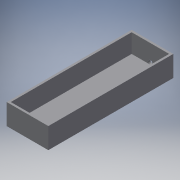
# Autodesk Inventor part: Trough
Saved by Autodesk Inventor 2019 (Build 230136000, 136)
## iProperties
Created: 2019-11-13
Part Number: Trough
Material: Generic
Document SubType Name: Modeling
Designer: Administrator
Density: 1 g/cm^3
Appearance: Default
Author: Administrator
Autodesk Inventor part; units mm, degrees
ref_plane "YZ Plane" through (0, 0, 0) normal (1, 0, 0) x (0, 1, 0)
ref_plane "XZ Plane" through (0, 0, 0) normal (0, 1, 0) x (-1, 0, 0)
ref_plane "XY Plane" through (0, 0, 0) normal (0, 0, 1) x (1, 0, 0)
sketch "Sketch1" plane through (0, 0, 0) normal (0, 1, 0) x (-1, 0, 0)
  line L0 (254, 762) -> (-254, 762)
  line L1 (-254, 762) -> (-254, -762)
  line L2 (-254, -762) -> (254, -762)
  line L3 (254, -762) -> (254, 762)
  line L4 (254, 762) -> (-254, -762) construction
  line L5 (-254, 762) -> (254, -762) construction
  point P0 (0, 0)
  dimension "d0" = 508
  dimension "d1" = 1524
  constraints: 12 end point, 2 midpoint, 2 parallel, 1 horizontal, 1 perpendicular
  measures "d0" distance of L2.end L1.end
  measures "d1" distance of L1.end L0.end
extrude "Extrusion1" add sketch "Sketch1" along normal blind 254
sketch "Sketch2" plane through (0, 254, 0) normal (0, 1, 0) x (1, 0, 0)
  line L0 (-254, -762) -> (254, -762) projected
  line L1 (254, 762) -> (-254, 762)
  line L2 (-254, 762) -> (-254, -762)
  line L3 (-254, -762) -> (254, -762)
  line L4 (254, -762) -> (254, 762)
  line L5 (254, 762) -> (-254, -762) construction
  line L6 (-254, 762) -> (254, -762) construction
  line L7 (0, -762) -> (0, -736.6)
  line L8 (-254, 762) -> (-254, -762) projected
  line L9 (-254, 0) -> (-228.6, 0)
  line L10 (228.6, 736.6) -> (-228.6, 736.6)
  line L11 (-228.6, 736.6) -> (-228.6, -736.6)
  line L12 (-228.6, -736.6) -> (228.6, -736.6)
  line L13 (228.6, -736.6) -> (228.6, 736.6)
  line L14 (228.6, 736.6) -> (-228.6, -736.6) construction
  line L15 (-228.6, 736.6) -> (228.6, -736.6) construction
  point P0 (0, 0)
  dimension "d4" = 25.4
  dimension "d5" = 25.4
  constraints: 28 end point, 6 midpoint, 4 parallel, 3 horizontal, 2 perpendicular, 1 vertical
  measures "d4" distance of L7.start L7.end
  measures "d5" distance of L9.start L9.end
extrude "Extrusion2" cut sketch "Sketch2" against normal blind 228.6 contours L12 L11 L10 L13
sketch "Sketch3" plane through (254, 0, -762) normal (0, 0, -1) x (-1, 0, 0)
  line L0 (25.4, 254) -> (482.6, 254) projected
  line L1 (254, 254) -> (254, 50.8) construction
  circle A0 centre (254, 50.8) radius 25.4
  point P0 (254, 0)
  dimension "d8" = 203.2
  dimension "d9" = 50.8
  constraints: 2 end point, 1 centre point, 1 coincident, 1 midpoint, 1 vertical
  measures "d8" distance of L1.start L1.end
  measures "d9" diameter of A0
extrude "Extrusion3" cut sketch "Sketch3" against normal blind 228.6
body "Solid1"
